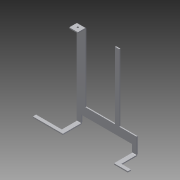
# Autodesk Inventor part: Puller Mechanism
Saved by Autodesk Inventor 2013 (Build 170138000, 138)
## iProperties
Created: 2013-01-28
Part Number: Puller Mechanism
Material: Aluminum 6061
Document SubType Name: Sheet Metal
Designer: Andrew Toennies
Density: 2.71 g/cm^3
Sheet Metal Rule: Default
Mass: 137.311 g
Surface Area: 374.947 cm^2
Volume: 50.6682 cm^3
Author: Andrew Toennies
Autodesk Inventor part; units mm, degrees
ref_plane "YZ Plane" through (0, 0, 0) normal (1, 0, 0) x (0, 1, 0)
ref_plane "XZ Plane" through (0, 0, 0) normal (0, 1, 0) x (-1, 0, 0)
ref_plane "XY Plane" through (0, 0, 0) normal (0, 0, 1) x (1, 0, 0)
sketch "Sketch5" plane through (0, -47.625, 57.15) normal (0, 1, 0) x (1, 0, 0)
  line L0 (0, 0) -> (0, 52.705)
  line L1 (176.53, 52.705) -> (163.83, 52.705)
  line L2 (163.83, 0) -> (163.83, 52.705)
  line L3 (163.83, 0) -> (176.53, 0)
  line L4 (176.53, 0) -> (176.53, 52.705)
  line L5 (0, 0) -> (-76.2, 0)
  line L6 (-76.2, 0) -> (-76.2, 9.525)
  line L7 (-76.2, 9.525) -> (0, 9.525)
  line L8 (176.53, 0) -> (205.105, 0)
  line L9 (205.105, 0) -> (205.105, 9.525)
  line L10 (205.105, 9.525) -> (176.53, 9.525)
  point P0 (0, 57.15)
  dimension "d37" = 76.2
  dimension "d38" = 9.525
  dimension "d39" = 28.575
  dimension "d40" = 9.525
  measures "d37" distance of L0.start L5.end
  measures "d38" distance of L5.end L6.end
  measures "d39" distance of L3.end L8.end
  measures "d40" distance of L8.end L9.end
sketch "Sketch7" plane through (0, 0, 3.175) normal (0, 0, 1) x (1, 0, 0)
  line L0 (25.4, 0) -> (176.53, 0)
  line L1 (125.73, 198.755) -> (125.73, 0)
  line L2 (176.53, 0) -> (176.53, -46.355)
  line L3 (125.73, 198.755) -> (113.03, 198.755)
  line L4 (113.03, 198.755) -> (113.03, 0)
  point P0 (0, 0)
  dimension "d60" = 12.7
  dimension "d61" = 50.8
  dimension "d62" = 198.755
  measures "d60" distance of L1.start L3.end
  measures "d61" distance between parallel lines of L1 L2
  measures "d62" distance between parallel lines of L0 L3
sketch "Sketch1" plane through (0, 0, 0) normal (0, 0, 1) x (1, 0, 0)
  line L0 (0, 0) -> (0, 203.2)
  line L1 (0, 203.2) -> (25.4, 203.2)
  line L2 (25.4, 203.2) -> (25.4, 0)
  line L3 (25.4, 0) -> (176.53, 0)
  line L4 (176.53, 0) -> (176.53, -25.4)
  line L5 (176.53, -25.4) -> (176.53, -50.8)
  line L6 (176.53, -50.8) -> (163.83, -50.8)
  line L7 (163.83, -50.8) -> (163.83, -25.4)
  line L8 (163.83, -25.4) -> (12.7, -25.4)
  line L9 (12.7, -25.4) -> (12.7, -50.8)
  line L10 (12.7, -50.8) -> (0, -50.8)
  line L11 (0, -50.8) -> (0, 0)
  line L12 (0, 0) -> (0, 0)
  dimension "d0" = 203.2
  dimension "d1" = 25.4
  dimension "d2" = 151.13
  dimension "d3" = 25.4
  dimension "d4" = 25.4
  dimension "d5" = 12.7
  dimension "d6" = 25.4
  dimension "d7" = 12.7
  dimension "d8" = 0
  dimension "d9" = 25.4
  dimension "d10" = 25.4
  measures "d0" distance of L0.start L0.end
  measures "d1" distance of L0.end L1.end
  measures "d2" distance of L2.end L3.end
  measures "d3" distance of L3.end L4.end
  measures "d4" distance of L4.end L5.end
  measures "d5" distance of L5.end L6.end
  measures "d6" distance of L8.end L9.end
  measures "d7" distance of L9.end L10.end
  measures "d8" distance of L11.end L0.start
  measures "d9" distance between parallel lines of L8 L3
  measures "d10" distance between parallel lines of L8 L12
extrude "Plate1" add sketch "Sketch1" along normal blind 3.175
sketch "Sketch2" plane through (12.7, -47.625, 0) normal (0, -1, 0) x (1, 0, 0)
  line L0 (-12.7, 0) -> (0, 0)
  line L1 (0, 0) -> (0, 57.15)
  line L2 (0, 57.15) -> (-12.7, 57.15)
  line L3 (-12.7, 57.15) -> (-12.7, 0)
  constraints: 6 end point, 1 horizontal, 1 perpendicular, 1 vertical
edge flange "Flange1" height 57.15 angle 90 thickness 3.175 bend radius 1.27 thickness toward (0, -1, 0) relief straight relief width 3.175 relief depth 1.5875 corner gap 3.175 corner form 0 edges at (6.35, -50.8, 3.175) (170.18, -50.8, 3.175) wall of the first edge with corners at (0, -47.625, 0) (12.7, -47.625, 0) (12.7, -47.625, 57.15) (0, -47.625, 57.15)
bend "Bend1"
corner "Corner1"
sketch "Sketch3" plane through (0, 200.025, 0) normal (0, 1, 0) x (-1, 0, 0)
  line L0 (-25.4, 0) -> (0, 0)
  line L1 (0, 0) -> (0, 25.4)
  line L2 (0, 25.4) -> (-25.4, 25.4)
  line L3 (-25.4, 25.4) -> (-25.4, 0)
  constraints: 6 end point, 1 horizontal, 1 perpendicular, 1 vertical
edge flange "Flange2" height 25.4 angle 90 thickness 3.175 bend radius 1.27 thickness toward (0, 1, 0) relief straight relief width 3.175 relief depth 1.5875 edges at (12.7, 203.2, 3.175) wall of the first edge with corners at (25.4, 200.025, 0) (0, 200.025, 0) (0, 200.025, 25.4) (25.4, 200.025, 25.4)
bend "Bend2"
corner "Corner2"
sketch "Sketch4" plane through (0, 203.2, 25.4) normal (0, 1, 0) x (1, 0, 0)
  line L0 (25.4, 0) -> (0, 0) projected
  line L1 (25.4, 20.955) -> (25.4, 0) projected
  circle A0 centre (12.7, 12.7) radius 2.413
  point P0 (0, 25.4)
  dimension "d32" = 4.826
  dimension "d33" = 12.7
  dimension "d34" = 12.7
  constraints: 1 centre point
  measures "d32" diameter of A0
  measures "d33" distance from line of L1 A0.centre
  measures "d34" distance from line of L0 A0.centre
extrude "Cut1" cut sketch "Sketch4" against normal blind 3.175
sheet face with bend "Face2" sketch "Sketch5" thickness 3.175 toward (0, -1, 0) bend radius 3.175 relief straight relief width 3.175 relief depth 1.5875 contours L5 L6 L7 L0 | L10 L9 L8 L4
bend "Bend3"
sheet face with bend "Face4" sketch "Sketch7" thickness 3.175 toward (0, 0, -1) bend radius 3.175 relief straight relief width 3.175 relief depth 1.5875
bend "Bend5"
equation "\"d35\" = Thickness"
equation "\"d12\" = BendReliefWidth"
equation "\"d13\" = BendReliefDepth"
equation "\"d14\" = MinimumRemnant"
equation "\"d15\" = BendRadius"
equation "\"d19\" = CornerReliefSize"
equation "\"d20\" = GapSize"
equation "\"d21\" = JacobiRadiusSize"
equation "\"d22\" = BendReliefWidth"
equation "\"d23\" = BendReliefDepth"
equation "\"d24\" = MinimumRemnant"
equation "\"d25\" = BendRadius"
equation "\"d29\" = CornerReliefSize"
equation "\"d30\" = GapSize"
equation "\"d31\" = JacobiRadiusSize"
equation "\"d41\" = BendRadius"
equation "\"d42\" = BendReliefWidth"
equation "\"d44\" = MinimumRemnant"
equation "\"d43\" = BendReliefDepth"
equation "\"d45\" = BendRadius"
equation "\"d55\" = BendRadius"
equation "\"d56\" = BendReliefWidth"
equation "\"d58\" = MinimumRemnant"
equation "\"d57\" = BendReliefDepth"
equation "\"d59\" = BendRadius"
equation "\"BendRadius\" = Thickness"
equation "\"BendReliefWidth\" = Thickness"
equation "\"BendReliefDepth\" = 0.5 * Thickness"
equation "\"CornerReliefSize\" = 4 * Thickness"
equation "\"MinimumRemnant\" = 2 * Thickness"
equation "\"TransitionRadius\" = BendRadius"
equation "\"JacobiRadiusSize\" = BendRadius"
equation "\"GapSize\" = Thickness"
equation "\"d11\" = BendRadius"
equation "\"Thickness\" = 3.175"
body "Solid1"
